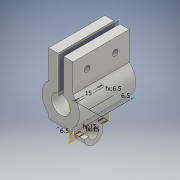
# Autodesk Inventor part: leverClamp
Saved by Autodesk Inventor 2018 (Build 220112000, 112)
## iProperties
Created: 2017-10-29
Part Number: leverClamp
Material: Generic
Document SubType Name: Modeling
Designer: Prakash
Density: 1 g/cm^3
Appearance: Default
Author: Prakash
Autodesk Inventor part; units mm, degrees
ref_plane "YZ Plane" through (0, 0, 0) normal (1, 0, 0) x (0, 1, 0)
ref_plane "XZ Plane" through (0, 0, 0) normal (0, 1, 0) x (-1, 0, 0)
ref_plane "XY Plane" through (0, 0, 0) normal (0, 0, 1) x (1, 0, 0)
sketch "Sketch1" plane through (0, 0, 0) normal (0, 1, 0) x (-1, 0, 0)
  arc A0 (5, -18) -> (5, -27.5394) centre (6.5, -22.7697) ccw
  line L0 (5, 0) -> (5, -18)
  line L1 (5, -27.5394) -> (5, -45.5394)
  line L2 (5, -18) -> (5, -27.5394) construction
  line L3 (5, -22.7697) -> (6.5, -22.7697) construction
  arc A1 (0, -15.1704) -> (0, -30.369) centre (6.5, -22.7697) ccw
  line L4 (0, 0) -> (0, -15.1704)
  line L5 (0, -30.369) -> (0, -45.5394)
  line L6 (5, 0) -> (0, 0)
  line L7 (0, -45.5394) -> (5, -45.5394)
  dimension "d0" = 10
  dimension "d1" = 1.5
  dimension "d2" = 5
  dimension "d4" = 5
  dimension "d5" = 18
  constraints: 16 end point, 5 point on circle, 3 coincident, 2 centre point, 2 collinear, 2 equal length, 2 horizontal, 2 vertical, 1 midpoint, 1 parallel
  measures "d0" diameter of A0
  measures "d1" distance of L3.start L3.end
  measures "d2" radial gap between concentric circles of A1 A0
  measures "d4" distance between parallel lines of L0 L4
  measures "d5" distance of L0.start L0.end
extrude "Extrusion1" add sketch "Sketch1" along normal blind 30
sketch "Sketch2" plane through (0, 0, 0) normal (1, 0, 0) x (0, 0, -1)
  line L0 (45.5394, 30) -> (27.5394, 30) projected
  line L1 (38.5394, 30) -> (38.5394, 0)
  line L2 (45.5394, 0) -> (45.5394, 30) projected
  line L3 (18, 30) -> (0, 30) projected
  line L4 (7, 30) -> (7, 0)
  line L5 (0, 0) -> (0, 30) projected
  line L6 (0, 0) -> (15.1704, 0) projected
  line L7 (30.369, 0) -> (45.5394, 0) projected
  point P0 (38.5394, 22.5)
  point P1 (38.5394, 7.5)
  point P2 (7, 22.5)
  point P3 (7, 7.5)
  dimension "d8" = 7
  dimension "d9" = 7
  dimension "d10" = 7.5
  dimension "d11" = 7.5
  dimension "d12" = 7.5
  dimension "d13" = 7.5
  dimension "d14" = 30
  dimension "d15" = 30
  constraints: 6 point on line, 4 end point, 2 vertical
  measures "d8" distance between parallel lines of L2 L1
  measures "d9" distance between parallel lines of L5 L4
  measures "d10" distance from line of L3 point (7, 22.5)
  measures "d11" distance from line of L6 point (7, 7.5)
  measures "d12" distance from line of L0 point (38.539, 22.5)
  measures "d13" distance from line of L7 point (38.539, 7.5)
  measures "d14" distance from line of L1.end L0
  measures "d15" distance from line of L4.end L0
hole "Hole1" at (0, 22.5, -7) at (0, 7.5, -7) direction (-1, 0, 0) diameter 3 end through all
ref_plane "Work Plane1" through (-6.5, 0, -18) normal (-1, 0, 0) x (0, 0, 1)
mirror "Mirror1" about plane through (-6.5, 0, -18) normal (-1, 0, 0) of "Extrusion1", "Hole1"
sketch "Sketch4" plane through (0, 30, 0) normal (0, 1, 0) x (1, 0, 0)
  arc A0 (-5, 18) -> (-5, 27.5394) centre (-6.5, 22.7697) ccw projected
  arc A1 (-8, 27.5394) -> (-8, 18) centre (-6.5, 22.7697) ccw projected
  arc A2 (-5, 27.5394) -> (-8, 27.5394) centre (-6.5, 22.7697) ccw
  line L0 (-5, 45.5394) -> (-5, 27.5394) projected
  line L1 (-8, 45.5394) -> (-8, 27.5394) projected
  line L2 (-5, 45.5394) -> (-8, 45.5394)
  line L3 (-5, 27.5394) -> (-5, 45.5394)
  line L4 (-8, 45.5394) -> (-8, 27.5394)
  point P0 (0, 0)
  constraints: 6 end point, 2 collinear, 2 point on circle, 1 centre point, 1 coincident, 1 concentric, 1 perpendicular
extrude "Extrusion2" add sketch "Sketch4" against normal up to surface (30 mm away)
sketch "Sketch5" plane through (0, 0, 0) normal (0, -1, 0) x (1, 0, 0)
  arc A0 (-8, -18) -> (-5, -18) centre (-6.5, -22.7697) ccw projected
  line L0 (-8, -18) -> (-8, 0) projected
  line L1 (-8, 0) -> (-13, 0) projected
  line L2 (-13, 0) -> (-13, -15.1704) projected
  arc A1 (-13, -15.1704) -> (-13, -30.369) centre (-6.5, -22.7697) ccw projected
  line L3 (-13, -30.369) -> (-13, -45.5394) projected
  line L4 (0, -45.5394) -> (-13, -45.5394) projected
  line L5 (0, -30.369) -> (0, -45.5394) projected
  arc A2 (0, -30.369) -> (0, -15.1704) centre (-6.5, -22.7697) ccw projected
  line L6 (0, 0) -> (0, -15.1704) projected
  line L7 (-5, 0) -> (0, 0) projected
  line L8 (-5, -18) -> (-5, 0) projected
  arc A3 (0, -30.369) -> (-13, -30.369) centre (-6.5, -22.7697) ccw
  line L9 (0, -30.369) -> (-13, -30.369)
  line L10 (-13, -30.369) -> (-13, -45.5394)
  line L11 (-13, -45.5394) -> (0, -45.5394)
  line L12 (0, -45.5394) -> (0, -30.369)
  arc A4 (-13, -30.369) -> (0, -30.369) centre (-6.5, -22.7697) ccw
  line L13 (0, -32.7697) -> (-13, -32.7697)
  constraints: 10 end point, 4 point on circle, 2 centre point, 2 parallel, 2 perpendicular, 2 point on line, 1 coincident, 1 horizontal, 1 tangent
extrude "Extrusion3" cut sketch "Sketch5" against normal up to surface (30 mm away) contours L13 L5 L4 L3
sketch "Sketch6" plane through (0, 0, -32.7697) normal (0, 0, -1) x (-1, 0, 0)
  line L0 (13, 15) -> (0, 15) construction
  line L1 (6.5, 30) -> (6.5, 0) construction
  point P0 (0, 0)
  point P1 (6.5, 15)
  dimension "d30" = 6.5
  dimension "d31" = 6.5
  dimension "d32" = 15
  dimension "d33" = 15
  dimension "d34" = 6.5
  dimension "d35" = 15
  constraints: 4 end point, 1 horizontal, 1 midpoint, 1 vertical
  measures "d30" distance from line of point (0, 0) L1
  measures "d31" distance from line of L0.start L1
  measures "d32" distance from line of L1.start L0
  measures "d33" distance from line of L1.end L0
  measures "d34" distance from line of L0.end L1
  measures "d35" distance from line of point (0, 0) L0
ref_plane "Work Plane2" through (-6.5, 15, -32.7697) normal (1, 0, 0) x (0, 1, 0)
sketch "Sketch7" plane through (-6.5, 15, -32.7697) normal (1, 0, 0) x (0, 1, 0)
  line L0 (-15, 0) -> (15, 0) projected
  line L1 (0, 0) -> (-2.5, 0)
  line L2 (-2.5, 0) -> (2.5, 0)
  line L3 (2.5, 0) -> (2.5, -5)
  line L4 (2.5, -5) -> (-2.5, -5)
  line L5 (-2.5, -5) -> (-2.5, 0)
  line L6 (0, 0) -> (0, -10)
  circle A0 centre (0, -10) radius 5
  circle A1 centre (0, -10) radius 2.5
  line L7 (2.5, -5) -> (2.5, -5.6699)
  line L8 (0, -10) -> (-1.118, -7.7639) construction
  line L9 (-1.118, -7.7639) -> (-2.5, -5)
  line L10 (0, -10) -> (-2.5, -10) construction
  line L11 (-2.5, -10) -> (-5, -10)
  point P0 (-15, 32.7697)
  dimension "d36" = 2.5
  dimension "d37" = 5
  dimension "d38" = 5
  dimension "d39" = 10
  dimension "d40" = 5
  constraints: 22 end point, 4 point on circle, 2 centre point, 2 coincident, 2 horizontal, 2 parallel, 2 point on line, 2 tangent, 1 collinear, 1 midpoint, 1 perpendicular, 1 vertical
  measures "d36" distance of L1.start L1.end
  measures "d37" distance of L1.end L2.end
  measures "d38" distance of L2.end L3.end
  measures "d39" distance of L1.start L6.end
  measures "d40" diameter of A1
extrude "Extrusion4" add sketch "Sketch7" along normal mid plane 5 contours L0 L6 L4 L5 | L0 L3 L4 L6 | L4 A0 L9 | A0 L11 A1 L6 | L4 L7 A0 | L6 A1 L9 A0
fillet "Fillet1" radius 4 4 edges at (-4, 15, -32.7697) (-6.5, 12.5, -32.7697) (-6.5, 17.5, -32.7697) (-9, 15, -32.7697)
equation "\"d11\" = d10"
equation "\"d12\" = d10"
equation "\"d13\" = d10"
equation "\"d31\" = d34"
equation "\"d33\" = d32"
equation "\"d35\" = d33"
body "Solid1"
